Autodesk Fusion 360 part; units mm, degrees
(part 4 of 7)
  spline S257 degree 3 poles (0.768, 12.1665) (0.7347, 12.1331) (0.6728, 12.1046) (0.6299, 12.1046) knots 0 0 0 0 1 1 1 1
  spline S258 degree 3 poles (0.6299, 12.1046) (0.5918, 12.1046) (0.4775, 12.0331) (0.3775, 11.9474) knots 0 0 0 0 1 1 1 1
  spline S259 degree 3 poles (0.3775, 11.9474) (0.2727, 11.8617) (0.1298, 11.7569) (0.0584, 11.7188) knots 0 0 0 0 1 1 1 1
  spline S260 degree 3 poles (0.0584, 11.7188) (-0.0131, 11.6855) (-0.175, 11.5807) (-0.294, 11.4997) knots 0 0 0 0 1 1 1 1
  spline S261 degree 3 poles (-0.294, 11.4997) (-0.5417, 11.3235) (-0.637, 11.3045) (-0.6131, 11.4283) knots 0 0 0 0 1 1 1 1
  spline S262 degree 3 poles (-0.6131, 11.4283) (-0.5989, 11.514) (-0.5179, 11.5664) (0.4584, 12.176) knots 0 0 0 0 1 1 1 1
  spline S263 degree 3 poles (-2.9087, 11.6283) (-3.0564, 11.6283) (-3.0992, 11.6474) (-3.0992, 11.714) knots 0 0 0 0 1 1 1 1
  spline S264 degree 3 poles (-3.0992, 11.714) (-3.0992, 11.7855) (-3.0325, 11.795) (-2.5372, 11.8093) knots 0 0 0 0 1 1 1 1
  spline S265 degree 3 poles (-2.5372, 11.8093) (-2.2324, 11.8141) (-1.9324, 11.8093) (-1.8705, 11.795) knots 0 0 0 0 1 1 1 1
  spline S266 degree 3 poles (-1.8705, 11.795) (-1.68, 11.7474) (-1.7514, 11.6378) (-1.9895, 11.6045) knots 0 0 0 0 1 1 1 1
  spline S267 degree 3 poles (-1.9895, 11.6045) (-2.2229, 11.5712) (-2.4801, 11.4045) (-2.4801, 11.2806) knots 0 0 0 0 1 1 1 1
  spline S268 degree 3 poles (-2.4801, 11.2806) (-2.4801, 11.2473) (-2.4991, 11.1997) (-2.5229, 11.1759) knots 0 0 0 0 1 1 1 1
  spline S269 degree 3 poles (-2.5229, 11.1759) (-2.5468, 11.1473) (-2.7182, 10.7949) (-2.8992, 10.39) knots 0 0 0 0 1 1 1 1
  spline S270 degree 3 poles (-2.8992, 10.39) (-3.2373, 9.6423) (-3.8279, 8.4659) (-3.9184, 8.3516) knots 0 0 0 0 1 1 1 1
  spline S271 degree 3 poles (-3.9184, 8.3516) (-3.9946, 8.2659) (-4.0279, 8.3135) (-4.2137, 8.7803) knots 0 0 0 0 1 1 1 1
  spline S272 degree 3 poles (-4.2137, 8.7803) (-4.3042, 9.0089) (-4.4423, 9.3137) (-4.5185, 9.4661) knots 0 0 0 0 1 1 1 1
  line L24 (-4.5185, 9.4661) -> (-4.6566, 9.7376)
  line L25 (-4.6566, 9.7376) -> (-4.7947, 9.4089)
  spline S273 degree 3 poles (-4.7947, 9.4089) (-4.8709, 9.228) (-4.9471, 9.0755) (-4.9662, 9.066) knots 0 0 0 0 1 1 1 1
  spline S274 degree 3 poles (-4.9662, 9.066) (-4.99, 9.0565) (-5.0043, 9.0232) (-5.0043, 8.9898) knots 0 0 0 0 1 1 1 1
  spline S275 degree 3 poles (-5.0043, 8.9898) (-5.0043, 8.8946) (-5.2091, 8.4183) (-5.2662, 8.3802) knots 0 0 0 0 1 1 1 1
  spline S276 degree 3 poles (-5.2662, 8.3802) (-5.3424, 8.3278) (-5.4091, 8.4326) (-5.552, 8.8184) knots 0 0 0 0 1 1 1 1
  spline S277 degree 3 poles (-5.552, 8.8184) (-5.7091, 9.2375) (-6.0187, 9.9804) (-6.2616, 10.4996) knots 0 0 0 0 1 1 1 1
  spline S278 degree 3 poles (-6.2616, 10.4996) (-6.3569, 10.6996) (-6.4331, 10.8806) (-6.4331, 10.8949) knots 0 0 0 0 1 1 1 1
  spline S279 degree 3 poles (-6.4331, 10.8949) (-6.4331, 10.9758) (-6.695, 11.5188) (-6.7617, 11.5712) knots 0 0 0 0 1 1 1 1
  spline S280 degree 3 poles (-6.7617, 11.5712) (-6.7998, 11.5997) (-6.895, 11.6283) (-6.9712, 11.6283) knots 0 0 0 0 1 1 1 1
  spline S281 degree 3 poles (-6.9712, 11.6283) (-7.057, 11.6283) (-7.0998, 11.6474) (-7.0903, 11.6902) knots 0 0 0 0 1 1 1 1
  spline S282 degree 3 poles (-7.0903, 11.6902) (-7.076, 11.7283) (-6.9093, 11.7521) (-6.5331, 11.7617) knots 0 0 0 0 1 1 1 1
  spline S283 degree 3 poles (-6.5331, 11.7617) (-6.0425, 11.7712) (-5.9997, 11.7664) (-6.0139, 11.6902) knots 0 0 0 0 1 1 1 1
  spline S284 degree 3 poles (-6.0139, 11.6902) (-6.0235, 11.6378) (-6.0854, 11.595) (-6.1711, 11.5807) knots 0 0 0 0 1 1 1 1
  spline S285 degree 3 poles (-6.1711, 11.5807) (-6.2473, 11.5664) (-6.3045, 11.5426) (-6.2997, 11.5235) knots 0 0 0 0 1 1 1 1
  spline S286 degree 3 poles (-6.2997, 11.5235) (-6.2521, 11.3711) (-6.214, 11.2806) (-6.0901, 11.0092) knots 0 0 0 0 1 1 1 1
  spline S287 degree 3 poles (-6.0901, 11.0092) (-6.0092, 10.8377) (-5.8806, 10.552) (-5.8044, 10.3662) knots 0 0 0 0 1 1 1 1
  spline S288 degree 3 poles (-5.8044, 10.3662) (-5.7282, 10.1852) (-5.6377, 9.99) (-5.6044, 9.9376) knots 0 0 0 0 1 1 1 1
  spline S289 degree 3 poles (-5.6044, 9.9376) (-5.571, 9.8852) (-5.5043, 9.7376) (-5.4615, 9.6042) knots 0 0 0 0 1 1 1 1
  spline S290 degree 3 poles (-5.4615, 9.6042) (-5.4186, 9.4756) (-5.3519, 9.3137) (-5.3186, 9.2518) knots 0 0 0 0 1 1 1 1
  line L26 (-5.3186, 9.2518) -> (-5.2519, 9.1327)
  line L27 (-5.2519, 9.1327) -> (-5.1614, 9.3232)
  spline S291 degree 3 poles (-5.1614, 9.3232) (-5.109, 9.4232) (-5.0281, 9.609) (-4.9852, 9.728) knots 0 0 0 0 1 1 1 1
  spline S292 degree 3 poles (-4.9852, 9.728) (-4.9043, 9.9423) (-4.9043, 9.9566) (-5.0043, 10.2043) knots 0 0 0 0 1 1 1 1
  spline S293 degree 3 poles (-5.0043, 10.2043) (-5.1948, 10.6663) (-5.2519, 10.7901) (-5.3615, 11.0092) knots 0 0 0 0 1 1 1 1
  spline S294 degree 3 poles (-5.3615, 11.0092) (-5.4186, 11.1282) (-5.4853, 11.2902) (-5.4996, 11.3759) knots 0 0 0 0 1 1 1 1
  spline S295 degree 3 poles (-5.4996, 11.3759) (-5.5377, 11.5426) (-5.5996, 11.6093) (-5.7377, 11.6331) knots 0 0 0 0 1 1 1 1
  spline S296 degree 3 poles (-5.7377, 11.6331) (-5.7901, 11.6426) (-5.8377, 11.6807) (-5.852, 11.714) knots 0 0 0 0 1 1 1 1
  spline S297 degree 3 poles (-5.852, 11.714) (-5.8663, 11.7569) (-5.7425, 11.7712) (-5.3377, 11.7712) knots 0 0 0 0 1 1 1 1
  spline S298 degree 3 poles (-5.3377, 11.7712) (-4.8566, 11.7712) (-4.809, 11.7617) (-4.8233, 11.6902) knots 0 0 0 0 1 1 1 1
  spline S299 degree 3 poles (-4.8233, 11.6902) (-4.8328, 11.6378) (-4.8947, 11.595) (-4.9805, 11.5807) knots 0 0 0 0 1 1 1 1
  spline S300 degree 3 poles (-4.9805, 11.5807) (-5.0567, 11.5664) (-5.1281, 11.5235) (-5.1376, 11.4807) knots 0 0 0 0 1 1 1 1
  spline S301 degree 3 poles (-5.1376, 11.4807) (-5.1424, 11.4426) (-5.0757, 11.2425) (-4.9805, 11.0377) knots 0 0 0 0 1 1 1 1
  spline S302 degree 3 poles (-4.9805, 11.0377) (-4.89, 10.8377) (-4.8138, 10.6472) (-4.8138, 10.6186) knots 0 0 0 0 1 1 1 1
  spline S303 degree 3 poles (-4.8138, 10.6186) (-4.8138, 10.5281) (-4.6614, 10.2472) (-4.6233, 10.271) knots 0 0 0 0 1 1 1 1
  spline S304 degree 3 poles (-4.6233, 10.271) (-4.5566, 10.3091) (-4.3851, 10.7187) (-4.3851, 10.8282) knots 0 0 0 0 1 1 1 1
  spline S305 degree 3 poles (-4.3851, 10.8282) (-4.3899, 10.8901) (-4.428, 11.0235) (-4.4804, 11.1282) knots 0 0 0 0 1 1 1 1
  spline S306 degree 3 poles (-4.4804, 11.1282) (-4.5328, 11.233) (-4.5709, 11.3664) (-4.5756, 11.4283) knots 0 0 0 0 1 1 1 1
  spline S307 degree 3 poles (-4.5756, 11.4283) (-4.5756, 11.4854) (-4.609, 11.5473) (-4.6471, 11.5616) knots 0 0 0 0 1 1 1 1
  spline S308 degree 3 poles (-4.6471, 11.5616) (-4.6852, 11.5807) (-4.7185, 11.6331) (-4.7185, 11.6807) knots 0 0 0 0 1 1 1 1
  spline S309 degree 3 poles (-4.7185, 11.6807) (-4.7185, 11.7664) (-4.6757, 11.7712) (-4.1708, 11.7712) knots 0 0 0 0 1 1 1 1
  spline S310 degree 3 poles (-4.1708, 11.7712) (-3.6803, 11.7712) (-3.6231, 11.7617) (-3.6231, 11.6902) knots 0 0 0 0 1 1 1 1
  spline S311 degree 3 poles (-3.6231, 11.6902) (-3.6231, 11.6188) (-3.666, 11.6045) (-3.9041, 11.6045) knots 0 0 0 0 1 1 1 1
  spline S312 degree 3 poles (-3.9041, 11.6045) (-4.0613, 11.6045) (-4.2042, 11.5854) (-4.2232, 11.5664) knots 0 0 0 0 1 1 1 1
  spline S313 degree 3 poles (-4.2232, 11.5664) (-4.247, 11.5473) (-4.2327, 11.4616) (-4.1994, 11.3759) knots 0 0 0 0 1 1 1 1
  spline S314 degree 3 poles (-4.1994, 11.3759) (-4.1661, 11.2902) (-4.066, 11.033) (-3.9803, 10.7949) knots 0 0 0 0 1 1 1 1
  spline S315 degree 3 poles (-3.9803, 10.7949) (-3.8946, 10.5615) (-3.7565, 10.2186) (-3.6755, 10.0376) knots 0 0 0 0 1 1 1 1
  spline S316 degree 3 poles (-3.6755, 10.0376) (-3.5279, 9.7137) (-3.5231, 9.709) (-3.4517, 9.8138) knots 0 0 0 0 1 1 1 1
  spline S317 degree 3 poles (-3.4517, 9.8138) (-3.4088, 9.8709) (-3.2945, 10.1138) (-3.1945, 10.3567) knots 0 0 0 0 1 1 1 1
  spline S318 degree 3 poles (-3.1945, 10.3567) (-3.0945, 10.5996) (-2.9468, 10.9473) (-2.8659, 11.1282) knots 0 0 0 0 1 1 1 1
  spline S319 degree 3 poles (-2.8659, 11.1282) (-2.6658, 11.5807) (-2.6706, 11.6283) (-2.9087, 11.6283) knots 0 0 0 0 1 1 1 1
  spline S320 degree 3 poles (0.387, 11.6331) (0.2679, 11.6807) (0.2727, 11.6807) (0.5489, 11.8664) knots 0 0 0 0 1 1 1 1
  spline S321 degree 3 poles (0.5489, 11.8664) (0.7013, 11.9712) (0.8442, 12.0569) (0.868, 12.0569) knots 0 0 0 0 1 1 1 1
  spline S322 degree 3 poles (0.868, 12.0569) (0.8871, 12.0569) (0.9014, 11.6188) (0.9014, 11.0806) knots 0 0 0 0 1 1 1 1
  spline S323 degree 3 poles (0.9014, 11.0806) (0.9014, 10.5424) (0.9109, 10.1043) (0.9157, 10.1043) knots 0 0 0 0 1 1 1 1
  spline S324 degree 3 poles (0.9157, 10.1043) (0.9252, 10.1043) (1.049, 10.2186) (1.1919, 10.3567) knots 0 0 0 0 1 1 1 1
  spline S325 degree 3 poles (1.1919, 10.3567) (1.3348, 10.4948) (1.511, 10.6567) (1.5919, 10.7187) knots 0 0 0 0 1 1 1 1
  spline S326 degree 3 poles (1.5919, 10.7187) (1.7062, 10.8044) (1.7205, 10.833) (1.6634, 10.8711) knots 0 0 0 0 1 1 1 1
  spline S327 degree 3 poles (1.6634, 10.8711) (1.6253, 10.8949) (1.4967, 10.9092) (1.3776, 10.8996) knots 0 0 0 0 1 1 1 1
  spline S328 degree 3 poles (1.3776, 10.8996) (1.2157, 10.8949) (1.1633, 10.9092) (1.1633, 10.9615) knots 0 0 0 0 1 1 1 1
  spline S329 degree 3 poles (1.1633, 10.9615) (1.1633, 11.0187) (1.2633, 11.0377) (1.7015, 11.0473) knots 0 0 0 0 1 1 1 1
  spline S330 degree 3 poles (1.7015, 11.0473) (2.2349, 11.0616) (2.2397, 11.0568) (2.2254, 10.9568) knots 0 0 0 0 1 1 1 1
  spline S331 degree 3 poles (2.2254, 10.9568) (2.2158, 10.8853) (2.1349, 10.8091) (2.0063, 10.7425) knots 0 0 0 0 1 1 1 1
  spline S332 degree 3 poles (2.0063, 10.7425) (1.5919, 10.5234) (1.049, 10.009) (1.2347, 10.009) knots 0 0 0 0 1 1 1 1
  spline S333 degree 3 poles (1.2347, 10.009) (1.2633, 10.009) (1.2824, 9.9662) (1.2824, 9.9185) knots 0 0 0 0 1 1 1 1
  spline S334 degree 3 poles (1.2824, 9.9185) (1.2824, 9.8661) (1.3014, 9.8185) (1.3252, 9.809) knots 0 0 0 0 1 1 1 1
  spline S335 degree 3 poles (1.3252, 9.809) (1.3491, 9.8042) (1.4538, 9.6661) (1.5634, 9.5089) knots 0 0 0 0 1 1 1 1
  spline S336 degree 3 poles (1.5634, 9.5089) (1.8682, 9.0708) (2.0301, 8.9136) (2.1682, 8.9136) knots 0 0 0 0 1 1 1 1
  line L28 (2.1682, 8.9136) -> (2.292, 8.9136)
  line L29 (2.292, 8.9136) -> (2.1444, 9.0803)
  spline S337 degree 3 poles (2.1444, 9.0803) (2.0682, 9.1708) (1.9777, 9.3375) (1.9444, 9.447) knots 0 0 0 0 1 1 1 1
  spline S338 degree 3 poles (1.9444, 9.447) (1.8729, 9.7233) (1.9158, 10.1852) (2.0349, 10.4234) knots 0 0 0 0 1 1 1 1
  spline S339 degree 3 poles (2.0349, 10.4234) (2.1492, 10.6424) (2.6159, 11.0377) (2.8159, 11.0806) knots 0 0 0 0 1 1 1 1
  spline S340 degree 3 poles (2.8159, 11.0806) (3.1779, 11.1616) (3.6399, 10.8472) (3.8066, 10.4091) knots 0 0 0 0 1 1 1 1
  spline S341 degree 3 poles (3.8066, 10.4091) (3.8589, 10.2662) (3.9018, 10.1281) (3.9018, 10.1043) knots 0 0 0 0 1 1 1 1
  spline S342 degree 3 poles (3.9018, 10.1043) (3.9018, 10.0757) (3.5494, 10.0519) (3.0826, 10.0471) knots 0 0 0 0 1 1 1 1
  line L30 (3.0826, 10.0471) -> (2.2587, 10.0328)
  line L31 (2.2587, 10.0328) -> (2.2444, 9.8947)
  spline S343 degree 3 poles (2.2444, 9.8947) (2.2111, 9.628) (2.2825, 9.4423) (2.4826, 9.247) knots 0 0 0 0 1 1 1 1
  spline S344 degree 3 poles (2.4826, 9.247) (2.8493, 8.8993) (3.1207, 8.885) (3.5922, 9.1994) knots 0 0 0 0 1 1 1 1
  spline S345 degree 3 poles (3.5922, 9.1994) (3.9161, 9.4137) (3.9494, 9.4232) (3.9494, 9.3042) knots 0 0 0 0 1 1 1 1
  spline S346 degree 3 poles (3.9494, 9.3042) (3.9494, 9.1613) (3.6589, 8.8612) (3.4065, 8.7422) knots 0 0 0 0 1 1 1 1
  spline S347 degree 3 poles (3.4065, 8.7422) (3.1827, 8.6374) (3.1065, 8.6279) (2.3587, 8.6279) knots 0 0 0 0 1 1 1 1
  line L32 (2.3587, 8.6279) -> (1.5586, 8.6279)
  line L33 (1.5586, 8.6279) -> (1.5872, 8.7755)
  spline S348 degree 3 poles (1.5872, 8.7755) (1.611, 8.9041) (1.5777, 8.9755) (1.3252, 9.3089) knots 0 0 0 0 1 1 1 1
  spline S349 degree 3 poles (1.3252, 9.3089) (1.1633, 9.5232) (1.0252, 9.7233) (1.0109, 9.7566) knots 0 0 0 0 1 1 1 1
  spline S350 degree 3 poles (1.0109, 9.7566) (0.9442, 9.9281) (0.9014, 9.7709) (0.9014, 9.347) knots 0 0 0 0 1 1 1 1
  line L34 (0.9014, 9.347) -> (0.9014, 8.8708)
  line L35 (0.9014, 8.8708) -> (1.1062, 8.8565)
  spline S351 degree 3 poles (1.1062, 8.8565) (1.2681, 8.8469) (1.3062, 8.8231) (1.3062, 8.7469) knots 0 0 0 0 1 1 1 1
  spline S352 degree 3 poles (1.3062, 8.7469) (1.3062, 8.6517) (1.2729, 8.6517) (-0.4798, 8.6517) knots 0 0 0 0 1 1 1 1
  line L36 (-0.4798, 8.6517) -> (-2.2658, 8.6517)
  line L37 (-2.2658, 8.6517) -> (-2.2801, 8.7612)
  spline S353 degree 3 poles (-2.2801, 8.7612) (-2.2943, 8.866) (-2.2991, 8.866) (-2.4944, 8.7136) knots 0 0 0 0 1 1 1 1
  spline S354 degree 3 poles (-2.4944, 8.7136) (-2.6992, 8.5517) (-3.0611, 8.2516) (-3.5231, 7.8468) knots 0 0 0 0 1 1 1 1
  spline S355 degree 3 poles (-3.5231, 7.8468) (-3.6707, 7.7182) (-4.1851, 7.2229) (-4.6709, 6.7466) knots 0 0 0 0 1 1 1 1
  spline S356 degree 3 poles (-4.6709, 6.7466) (-5.5377, 5.8894) (-5.7663, 5.7131) (-5.7663, 5.9037) knots 0 0 0 0 1 1 1 1
  spline S357 degree 3 poles (-5.7663, 5.9037) (-5.7663, 5.956) (-5.5567, 6.1846) (-5.2519, 6.4704) knots 0 0 0 0 1 1 1 1
  spline S358 degree 3 poles (-5.2519, 6.4704) (-4.79, 6.9038) (-4.3661, 7.2753) (-2.742, 8.6993) knots 0 0 0 0 1 1 1 1
  spline S359 degree 3 poles (-2.742, 8.6993) (-2.442, 8.9612) (-2.0848, 9.3089) (-1.9467, 9.4708) knots 0 0 0 0 1 1 1 1
  spline S360 degree 3 poles (-1.9467, 9.4708) (-1.8086, 9.6328) (-1.4418, 10.0281) (-1.1323, 10.3567) knots 0 0 0 0 1 1 1 1
  spline S361 degree 3 poles (-1.1323, 10.3567) (-0.8275, 10.6805) (-0.575, 10.9711) (-0.575, 11.0044) knots 0 0 0 0 1 1 1 1
  spline S362 degree 3 poles (-0.575, 11.0044) (-0.575, 11.0377) (-0.7179, 11.0568) (-1.0132, 11.0568) knots 0 0 0 0 1 1 1 1
  spline S363 degree 3 poles (-1.0132, 11.0568) (-1.3513, 11.0568) (-1.4657, 11.0377) (-1.5371, 10.9758) knots 0 0 0 0 1 1 1 1
  spline S364 degree 3 poles (-1.5371, 10.9758) (-1.5847, 10.933) (-1.6704, 10.8758) (-1.7276, 10.8472) knots 0 0 0 0 1 1 1 1
  spline S365 degree 3 poles (-1.7276, 10.8472) (-1.7847, 10.8187) (-1.8752, 10.7044) (-1.9324, 10.5901) knots 0 0 0 0 1 1 1 1
  spline S366 degree 3 poles (-1.9324, 10.5901) (-2.0276, 10.3948) (-2.1467, 10.3186) (-2.1467, 10.4615) knots 0 0 0 0 1 1 1 1
  spline S367 degree 3 poles (-2.1467, 10.4615) (-2.1467, 10.4996) (-2.1229, 10.6329) (-2.0896, 10.7568) knots 0 0 0 0 1 1 1 1
  spline S368 degree 3 poles (-2.0896, 10.7568) (-2.061, 10.8853) (-2.0181, 11.0711) (-1.9943, 11.1711) knots 0 0 0 0 1 1 1 1
  line L38 (-1.9943, 11.1711) -> (-1.9467, 11.3568)
  line L39 (-1.9467, 11.3568) -> (-1.0465, 11.3283)
  spline S369 degree 3 poles (-1.0465, 11.3283) (-0.4988, 11.3092) (-0.1369, 11.3187) (-0.1226, 11.3473) knots 0 0 0 0 1 1 1 1
  spline S370 degree 3 poles (-0.1226, 11.3473) (-0.0893, 11.3997) (0.0012, 11.4045) (0.0822, 11.3473) knots 0 0 0 0 1 1 1 1
  spline S371 degree 3 poles (0.0822, 11.3473) (0.206, 11.2711) (0.0774, 11.0616) (-0.3464, 10.6424) knots 0 0 0 0 1 1 1 1
  spline S372 degree 3 poles (-0.3464, 10.6424) (-0.5798, 10.4138) (-1.0418, 9.9376) (-1.3704, 9.5899) knots 0 0 0 0 1 1 1 1
  line L40 (-1.3704, 9.5899) -> (-1.9705, 8.9612)
  line L41 (-1.9705, 8.9612) -> (-1.0227, 8.9708)
  line L42 (-1.0227, 8.9708) -> (-0.0797, 8.9851)
  line L43 (-0.0797, 8.9851) -> (-0.0369, 9.1756)
  spline S373 degree 3 poles (-0.0369, 9.1756) (0.0203, 9.4137) (0.025, 9.4185) (0.1155, 9.328) knots 0 0 0 0 1 1 1 1
  spline S374 degree 3 poles (0.1155, 9.328) (0.1584, 9.2851) (0.187, 9.1708) (0.187, 9.0565) knots 0 0 0 0 1 1 1 1
  spline S375 degree 3 poles (0.187, 9.0565) (0.187, 8.866) (0.1917, 8.8612) (0.3394, 8.8755) knots 0 0 0 0 1 1 1 1
  spline S376 degree 3 poles (0.3394, 8.8755) (0.4727, 8.8898) (0.4965, 8.9136) (0.5299, 9.0565) knots 0 0 0 0 1 1 1 1
  spline S377 degree 3 poles (0.5299, 9.0565) (0.5727, 9.247) (0.5775, 10.8377) (0.5346, 11.2854) knots 0 0 0 0 1 1 1 1
  spline S378 degree 3 poles (0.5346, 11.2854) (0.5108, 11.5521) (0.4965, 11.595) (0.387, 11.6331) knots 0 0 0 0 1 1 1 1
  spline S379 degree 3 poles (4.4876, 11.052) (4.6924, 11.0568) (4.7115, 11.0473) (4.7115, 10.9425) knots 0 0 0 0 1 1 1 1
  spline S380 degree 3 poles (4.7115, 10.9425) (4.7115, 10.7758) (4.7972, 10.7425) (4.9162, 10.8568) knots 0 0 0 0 1 1 1 1
  spline S381 degree 3 poles (4.9162, 10.8568) (5.183, 11.1044) (5.4973, 11.1663) (5.7878, 11.0282) knots 0 0 0 0 1 1 1 1
  spline S382 degree 3 poles (5.7878, 11.0282) (5.8783, 10.9854) (6.0164, 10.8711) (6.0926, 10.7758) knots 0 0 0 0 1 1 1 1
  line L44 (6.0926, 10.7758) -> (6.2355, 10.6043)
  line L45 (6.2355, 10.6043) -> (6.2403, 9.8423)
  spline S383 degree 3 poles (6.2403, 9.8423) (6.245, 8.9136) (6.2593, 8.8469) (6.4641, 8.8279) knots 0 0 0 0 1 1 1 1
  spline S384 degree 3 poles (6.4641, 8.8279) (6.5784, 8.8184) (6.6165, 8.7898) (6.6165, 8.7184) knots 0 0 0 0 1 1 1 1
  spline S385 degree 3 poles (6.6165, 8.7184) (6.6165, 8.6326) (6.5784, 8.6279) (6.045, 8.6279) knots 0 0 0 0 1 1 1 1
  spline S386 degree 3 poles (6.045, 8.6279) (5.7307, 8.6279) (5.4735, 8.6422) (5.4735, 8.666) knots 0 0 0 0 1 1 1 1
  spline S387 degree 3 poles (5.4735, 8.666) (5.4782, 8.7565) (5.5592, 8.8136) (5.7116, 8.8279) knots 0 0 0 0 1 1 1 1
  line L46 (5.7116, 8.8279) -> (5.8783, 8.8422)
  line L47 (5.8783, 8.8422) -> (5.8783, 9.6899)
  spline S388 degree 3 poles (5.8783, 9.6899) (5.8783, 10.4519) (5.8688, 10.5424) (5.7973, 10.5853) knots 0 0 0 0 1 1 1 1
  spline S389 degree 3 poles (5.7973, 10.5853) (5.7497, 10.6139) (5.7116, 10.6615) (5.7116, 10.6996) knots 0 0 0 0 1 1 1 1
  spline S390 degree 3 poles (5.7116, 10.6996) (5.7116, 10.7806) (5.4068, 10.8853) (5.2592, 10.8472) knots 0 0 0 0 1 1 1 1
  spline S391 degree 3 poles (5.2592, 10.8472) (5.202, 10.833) (5.0591, 10.7615) (4.9543, 10.6901) knots 0 0 0 0 1 1 1 1
  line L48 (4.9543, 10.6901) -> (4.7591, 10.5615)
  line L49 (4.7591, 10.5615) -> (4.7686, 9.7042)
  line L50 (4.7686, 9.7042) -> (4.7829, 8.8422)
  line L51 (4.7829, 8.8422) -> (4.9258, 8.8279)
  spline S392 degree 3 poles (4.9258, 8.8279) (5.0687, 8.8088) (5.1544, 8.7374) (5.1115, 8.666) knots 0 0 0 0 1 1 1 1
  spline S393 degree 3 poles (5.1115, 8.666) (5.0877, 8.6279) (3.9494, 8.6088) (3.9494, 8.6469) knots 0 0 0 0 1 1 1 1
  spline S394 degree 3 poles (3.9494, 8.6469) (3.9494, 8.7565) (4.0304, 8.8184) (4.1638, 8.8184) knots 0 0 0 0 1 1 1 1
  spline S395 degree 3 poles (4.1638, 8.8184) (4.2638, 8.8184) (4.3304, 8.8469) (4.3495, 8.8946) knots 0 0 0 0 1 1 1 1
  spline S396 degree 3 poles (4.3495, 8.8946) (4.3876, 8.9946) (4.3876, 10.4805) (4.3495, 10.671) knots 0 0 0 0 1 1 1 1
  spline S397 degree 3 poles (4.3495, 10.671) (4.3257, 10.7853) (4.2876, 10.8282) (4.178, 10.8568) knots 0 0 0 0 1 1 1 1
  spline S398 degree 3 poles (4.178, 10.8568) (3.8875, 10.9282) (4.0637, 11.0425) (4.4876, 11.052) knots 0 0 0 0 1 1 1 1
  circle A0 centre (0, 0) radius 14.0811
  spline S399 degree 3 poles (-5.2833, -10.8985) (-5.4134, -10.9708) (-5.5435, -11.0141) (-5.5724, -10.9925) knots 0 0 0 0 1 1 1 1
  spline S400 degree 3 poles (-5.5724, -10.9925) (-5.6013, -10.978) (-5.7024, -11.0069) (-5.8036, -11.0647) knots 0 0 0 0 1 1 1 1
  spline S401 degree 3 poles (-5.8036, -11.0647) (-6.0348, -11.1875) (-6.0348, -11.1875) (-5.9842, -11.0214) knots 0 0 0 0 1 1 1 1
  spline S402 degree 3 poles (-5.9842, -11.0214) (-5.9264, -10.8407) (-6.1359, -10.819) (-6.3527, -10.9852) knots 0 0 0 0 1 1 1 1
  spline S403 degree 3 poles (-6.3527, -10.9852) (-6.5333, -11.1225) (-7.0319, -11.1225) (-7.2342, -10.978) knots 0 0 0 0 1 1 1 1
  spline S404 degree 3 poles (-7.2342, -10.978) (-7.3859, -10.8769) (-7.3931, -10.819) (-7.3931, -9.8436) knots 0 0 0 0 1 1 1 1
  spline S405 degree 3 poles (-7.3931, -9.8436) (-7.3931, -9.0488) (-7.4148, -8.7815) (-7.5015, -8.6587) knots 0 0 0 0 1 1 1 1
  spline S406 degree 3 poles (-7.5015, -8.6587) (-7.5955, -8.5214) (-7.5955, -8.5069) (-7.4437, -8.4636) knots 0 0 0 0 1 1 1 1
  spline S407 degree 3 poles (-7.4437, -8.4636) (-7.227, -8.4058) (-6.7067, -8.4058) (-6.6489, -8.4708) knots 0 0 0 0 1 1 1 1
  spline S408 degree 3 poles (-6.6489, -8.4708) (-6.62, -8.4925) (-6.6851, -8.5936) (-6.7862, -8.6876) knots 0 0 0 0 1 1 1 1
  spline S409 degree 3 poles (-6.7862, -8.6876) (-6.9741, -8.861) (-6.9741, -8.8754) (-6.9452, -9.7208) knots 0 0 0 0 1 1 1 1
  spline S410 degree 3 poles (-6.9452, -9.7208) (-6.9235, -10.2844) (-6.8801, -10.6167) (-6.8223, -10.689) knots 0 0 0 0 1 1 1 1
  spline S411 degree 3 poles (-6.8223, -10.689) (-6.7212, -10.8118) (-6.4755, -10.8335) (-6.0998, -10.7612) knots 0 0 0 0 1 1 1 1
  line L52 (-6.0998, -10.7612) -> (-5.8758, -10.7179)
  line L53 (-5.8758, -10.7179) -> (-5.8758, -8.7093)
  line L54 (-5.8758, -8.7093) -> (-6.0781, -8.6225)
  line L55 (-6.0781, -8.6225) -> (-6.2732, -8.5431)
  line L56 (-6.2732, -8.5431) -> (-6.0565, -8.4853)
  spline S412 degree 3 poles (-6.0565, -8.4853) (-5.9408, -8.4491) (-5.6518, -8.4275) (-5.4206, -8.4347) knots 0 0 0 0 1 1 1 1
  line L57 (-5.4206, -8.4347) -> (-5.0016, -8.4419)
  line L58 (-5.0016, -8.4419) -> (-5.1894, -8.5936)
  spline S413 degree 3 poles (-5.1894, -8.5936) (-5.3773, -8.7454) (-5.3845, -8.7743) (-5.4206, -9.7352) knots 0 0 0 0 1 1 1 1
  line L59 (-5.4206, -9.7352) -> (-5.464, -10.7179)
  line L60 (-5.464, -10.7179) -> (-5.2544, -10.7468)
  line L61 (-5.2544, -10.7468) -> (-5.0449, -10.7685)
  line L62 (-5.0449, -10.7685) -> (-5.2833, -10.8985)
  spline S414 degree 3 poles (6.0388, -10.1399) (6.4289, -11.2742) (6.5662, -11.5271) (6.7541, -11.5271) knots 0 0 0 0 1 1 1 1
  spline S415 degree 3 poles (6.7541, -11.5271) (6.8624, -11.5271) (6.8624, -11.5416) (6.7685, -11.5994) knots 0 0 0 0 1 1 1 1
  spline S416 degree 3 poles (6.7685, -11.5994) (6.6312, -11.6861) (5.6341, -11.6933) (5.5836, -11.6066) knots 0 0 0 0 1 1 1 1
  spline S417 degree 3 poles (5.5836, -11.6066) (5.5619, -11.5705) (5.6052, -11.5271) (5.6847, -11.5055) knots 0 0 0 0 1 1 1 1
  spline S418 degree 3 poles (5.6847, -11.5055) (5.8003, -11.4766) (5.8292, -11.4043) (5.8292, -11.1948) knots 0 0 0 0 1 1 1 1
  spline S419 degree 3 poles (5.8292, -11.1948) (5.8292, -10.9347) (5.3018, -9.2439) (5.1862, -9.1211) knots 0 0 0 0 1 1 1 1
  spline S420 degree 3 poles (5.1862, -9.1211) (5.1067, -9.0416) (4.8321, -9.6341) (4.7382, -10.0893) knots 0 0 0 0 1 1 1 1
  spline S421 degree 3 poles (4.7382, -10.0893) (4.6154, -10.6673) (4.8683, -11.491) (5.1934, -11.5416) knots 0 0 0 0 1 1 1 1
  spline S422 degree 3 poles (5.1934, -11.5416) (5.3524, -11.5705) (5.3451, -11.5777) (5.1573, -11.6283) knots 0 0 0 0 1 1 1 1
  spline S423 degree 3 poles (5.1573, -11.6283) (5.0489, -11.6644) (4.6732, -11.6644) (4.3264, -11.6355) knots 0 0 0 0 1 1 1 1
  spline S424 degree 3 poles (4.3264, -11.6355) (3.8206, -11.5922) (3.7339, -11.5705) (3.8784, -11.5127) knots 0 0 0 0 1 1 1 1
  spline S425 degree 3 poles (3.8784, -11.5127) (4.2324, -11.3826) (4.3191, -11.2381) (4.2686, -10.8841) knots 0 0 0 0 1 1 1 1
  spline S426 degree 3 poles (4.2686, -10.8841) (4.218, -10.5373) (3.9362, -9.6919) (3.7556, -9.3306) knots 0 0 0 0 1 1 1 1
  line L63 (3.7556, -9.3306) -> (3.6472, -9.1283)
  line L64 (3.6472, -9.1283) -> (3.5316, -9.2945)
  spline S427 degree 3 poles (3.5316, -9.2945) (3.4738, -9.3812) (3.2498, -9.9014) (3.0475, -10.4361) knots 0 0 0 0 1 1 1 1
  spline S428 degree 3 poles (3.0475, -10.4361) (2.6356, -11.5127) (2.6356, -11.5055) (3.1559, -11.5344) knots 0 0 0 0 1 1 1 1
  spline S429 degree 3 poles (3.1559, -11.5344) (3.4015, -11.5416) (3.4015, -11.5488) (3.0836, -11.6066) knots 0 0 0 0 1 1 1 1
  spline S430 degree 3 poles (3.0836, -11.6066) (2.903, -11.6355) (2.5128, -11.6644) (2.2166, -11.6644) knots 0 0 0 0 1 1 1 1
  line L65 (2.2166, -11.6644) -> (1.6747, -11.6716)
  line L66 (1.6747, -11.6716) -> (1.9564, -11.5055)
  spline S431 degree 3 poles (1.9564, -11.5055) (2.2527, -11.332) (2.5056, -10.8913) (3.3004, -9.1283) knots 0 0 0 0 1 1 1 1
  spline S432 degree 3 poles (3.3004, -9.1283) (3.5099, -8.6587) (3.705, -8.2757) (3.7339, -8.2757) knots 0 0 0 0 1 1 1 1
  spline S433 degree 3 poles (3.7339, -8.2757) (3.7628, -8.2757) (3.9073, -8.5431) (4.0518, -8.8754) knots 0 0 0 0 1 1 1 1
  spline S434 degree 3 poles (4.0518, -8.8754) (4.5431, -9.9881) (4.5648, -10.0026) (4.7454, -9.4173) knots 0 0 0 0 1 1 1 1
  spline S435 degree 3 poles (4.7454, -9.4173) (4.9116, -8.9043) (5.1862, -8.2757) (5.2512, -8.2757) knots 0 0 0 0 1 1 1 1
  spline S436 degree 3 poles (5.2512, -8.2757) (5.3307, -8.2757) (5.6414, -9.0055) (6.0388, -10.1399) knots 0 0 0 0 1 1 1 1
  spline S437 degree 3 poles (-3.1735, -8.6587) (-2.6244, -9.085) (-2.4366, -10.0459) (-2.8267, -10.4795) knots 0 0 0 0 1 1 1 1
  spline S438 degree 3 poles (-2.8267, -10.4795) (-3.123, -10.819) (-3.3108, -10.9563) (-3.6143, -11.0647) knots 0 0 0 0 1 1 1 1
  spline S439 degree 3 poles (-3.6143, -11.0647) (-3.9539, -11.1803) (-4.055, -11.1875) (-4.3657, -11.0864) knots 0 0 0 0 1 1 1 1
  spline S440 degree 3 poles (-4.3657, -11.0864) (-4.6692, -10.9852) (-4.9365, -10.7468) (-4.9365, -10.5878) knots 0 0 0 0 1 1 1 1
  spline S441 degree 3 poles (-4.9365, -10.5878) (-4.9365, -10.3422) (-4.6764, -10.2121) (-4.055, -10.1471) knots 0 0 0 0 1 1 1 1
  spline S442 degree 3 poles (-4.055, -10.1471) (-3.0218, -10.0315) (-3.0363, -10.0387) (-3.0868, -9.7208) knots 0 0 0 0 1 1 1 1
  spline S443 degree 3 poles (-3.0868, -9.7208) (-3.1952, -9.0127) (-3.4264, -8.8176) (-4.1128, -8.8249) knots 0 0 0 0 1 1 1 1
  spline S444 degree 3 poles (-4.1128, -8.8249) (-4.4308, -8.8249) (-4.6331, -8.8754) (-4.8209, -8.9838) knots 0 0 0 0 1 1 1 1
  spline S445 degree 3 poles (-4.8209, -8.9838) (-5.1388, -9.1717) (-5.1605, -9.085) (-4.8643, -8.796) knots 0 0 0 0 1 1 1 1
  spline S446 degree 3 poles (-4.8643, -8.796) (-4.4308, -8.3624) (-3.6504, -8.2974) (-3.1735, -8.6587) knots 0 0 0 0 1 1 1 1
  spline S447 degree 3 poles (1.9131, -10.4578) (1.9564, -10.978) (1.8914, -11.0141) (0.8943, -11.043) knots 0 0 0 0 1 1 1 1
  spline S448 degree 3 poles (0.8943, -11.043) (0.4102, -11.0503) (-0.0594, -11.0719) (-0.1461, -11.0792) knots 0 0 0 0 1 1 1 1
  spline S449 degree 3 poles (-0.1461, -11.0792) (-0.2328, -11.0864) (-0.3195, -11.0647) (-0.3484, -11.0286) knots 0 0 0 0 1 1 1 1
  spline S450 degree 3 poles (-0.3484, -11.0286) (-0.3701, -10.9925) (-0.0667, -10.5589) (0.3235, -10.0676) knots 0 0 0 0 1 1 1 1
  spline S451 degree 3 poles (0.3235, -10.0676) (0.7137, -9.5763) (1.1255, -9.0561) (1.2339, -8.9116) knots 0 0 0 0 1 1 1 1
  line L67 (1.2339, -8.9116) -> (1.4362, -8.637)
  line L68 (1.4362, -8.637) -> (0.8654, -8.637)
  spline S452 degree 3 poles (0.8654, -8.637) (0.2151, -8.637) (0.0562, -8.7165) (-0.1678, -9.1283) knots 0 0 0 0 1 1 1 1
  spline S453 degree 3 poles (-0.1678, -9.1283) (-0.2906, -9.374) (-0.3051, -9.3812) (-0.3123, -9.215) knots 0 0 0 0 1 1 1 1
  spline S454 degree 3 poles (-0.3123, -9.215) (-0.3123, -9.1139) (-0.2545, -8.8971) (-0.1895, -8.7309) knots 0 0 0 0 1 1 1 1
  line L69 (-0.1895, -8.7309) -> (-0.0594, -8.4202)
  line L70 (-0.0594, -8.4202) -> (1.075, -8.4202)
  spline S455 degree 3 poles (1.075, -8.4202) (1.8914, -8.4202) (2.2166, -8.4419) (2.2166, -8.5069) knots 0 0 0 0 1 1 1 1
  spline S456 degree 3 poles (2.2166, -8.5069) (2.2166, -8.6153) (1.7469, -9.215) (1.0027, -10.0676) knots 0 0 0 0 1 1 1 1
  spline S457 degree 3 poles (1.0027, -10.0676) (0.3163, -10.8552) (0.3235, -10.8985) (1.0894, -10.8263) knots 0 0 0 0 1 1 1 1
  spline S458 degree 3 poles (1.0894, -10.8263) (1.5663, -10.7829) (1.5735, -10.7757) (1.7325, -10.4867) knots 0 0 0 0 1 1 1 1
  line L71 (1.7325, -10.4867) -> (1.8914, -10.1904)
  line L72 (1.8914, -10.1904) -> (1.9131, -10.4578)
  spline S459 degree 3 poles (-0.4279, -11.7078) (-0.1245, -11.7945) (-0.1389, -11.8378) (-0.4929, -11.9173) knots 0 0 0 0 1 1 1 1
  spline S460 degree 3 poles (-0.4929, -11.9173) (-0.7675, -11.9896) (-0.8903, -12.0907) (-0.8903, -12.2569) knots 0 0 0 0 1 1 1 1
  spline S461 degree 3 poles (-0.8903, -12.2569) (-0.8903, -12.4086) (-1.071, -12.4447) (-1.1505, -12.3075) knots 0 0 0 0 1 1 1 1
  spline S462 degree 3 poles (-1.1505, -12.3075) (-1.1794, -12.2641) (-1.1938, -11.6572) (-1.1866, -10.9708) knots 0 0 0 0 1 1 1 1
  line L73 (-1.1866, -10.9708) -> (-1.1721, -9.7136)
  line L74 (-1.1721, -9.7136) -> (-1.3455, -9.8292)
  spline S463 degree 3 poles (-1.3455, -9.8292) (-1.4395, -9.887) (-1.6707, -10.1326) (-1.8513, -10.3711) knots 0 0 0 0 1 1 1 1
  line L75 (-1.8513, -10.3711) -> (-2.1837, -10.7974)
  line L76 (-2.1837, -10.7974) -> (-1.9236, -10.819)
  spline S464 degree 3 poles (-1.9236, -10.819) (-1.7791, -10.8335) (-1.649, -10.8841) (-1.6273, -10.9347) knots 0 0 0 0 1 1 1 1
  spline S465 degree 3 poles (-1.6273, -10.9347) (-1.6056, -10.9997) (-1.7502, -11.0214) (-2.1837, -11.0214) knots 0 0 0 0 1 1 1 1
  spline S466 degree 3 poles (-2.1837, -11.0214) (-2.5088, -11.0214) (-2.7689, -10.9925) (-2.7689, -10.9563) knots 0 0 0 0 1 1 1 1
  spline S467 degree 3 poles (-2.7689, -10.9563) (-2.7689, -10.9202) (-2.5883, -10.7323) (-2.3715, -10.5517) knots 0 0 0 0 1 1 1 1
  spline S468 degree 3 poles (-2.3715, -10.5517) (-2.1548, -10.3639) (-1.9958, -10.1832) (-2.0175, -10.1471) knots 0 0 0 0 1 1 1 1
  spline S469 degree 3 poles (-2.0175, -10.1471) (-2.0392, -10.111) (-2.0175, -10.0893) (-1.9669, -10.0965) knots 0 0 0 0 1 1 1 1
  spline S470 degree 3 poles (-1.9669, -10.0965) (-1.9163, -10.111) (-1.8296, -10.0315) (-1.7646, -9.9231) knots 0 0 0 0 1 1 1 1
  spline S471 degree 3 poles (-1.7646, -9.9231) (-1.649, -9.728) (-1.649, -9.7208) (-2.1186, -9.2439) knots 0 0 0 0 1 1 1 1
  spline S472 degree 3 poles (-2.1186, -9.2439) (-2.3788, -8.9838) (-2.7183, -8.702) (-2.8773, -8.6153) knots 0 0 0 0 1 1 1 1
  line L77 (-2.8773, -8.6153) -> (-3.1663, -8.4564)
  line L78 (-3.1663, -8.4564) -> (-2.5955, -8.4347)
  spline S473 degree 3 poles (-2.5955, -8.4347) (-1.9814, -8.413) (-1.9091, -8.4347) (-2.0392, -8.5936) knots 0 0 0 0 1 1 1 1
  spline S474 degree 3 poles (-2.0392, -8.5936) (-2.1042, -8.6731) (-2.0319, -8.7743) (-1.6707, -9.1283) knots 0 0 0 0 1 1 1 1
  line L79 (-1.6707, -9.1283) -> (-1.2155, -9.5691)
  line L80 (-1.2155, -9.5691) -> (-1.1721, -9.3306)
  spline S475 degree 3 poles (-1.1721, -9.3306) (-1.0999, -8.8899) (-1.1721, -8.5936) (-1.3817, -8.5142) knots 0 0 0 0 1 1 1 1
  spline S476 degree 3 poles (-1.3817, -8.5142) (-1.5478, -8.4491) (-1.4756, -8.4347) (-0.9843, -8.4275) knots 0 0 0 0 1 1 1 1
  spline S477 degree 3 poles (-0.9843, -8.4275) (-0.399, -8.4202) (-0.1967, -8.4997) (-0.5652, -8.5936) knots 0 0 0 0 1 1 1 1
  line L81 (-0.5652, -8.5936) -> (-0.7458, -8.637)
  line L82 (-0.7458, -8.637) -> (-0.7314, -10.1326)
  line L83 (-0.7314, -10.1326) -> (-0.7097, -11.6283)
  line L84 (-0.7097, -11.6283) -> (-0.4279, -11.7078)
  spline S478 degree 3 poles (3.2862, -4.7869) (3.2932, -4.78) (3.4519, -4.7635) (3.5898, -4.7557) knots 0 0 0 0 1 1 1 1
  spline S479 degree 3 poles (3.5898, -4.7557) (3.6592, -4.7523) (3.739, -4.7427) (3.7676, -4.7358) knots 0 0 0 0 1 1 1 1
  spline S480 degree 3 poles (3.7676, -4.7358) (3.7963, -4.728) (3.8466, -4.7184) (3.8804, -4.7132) knots 0 0 0 0 1 1 1 1
  spline S481 degree 3 poles (3.8804, -4.7132) (4.027, -4.6915) (4.2742, -4.6213) (4.3028, -4.5926) knots 0 0 0 0 1 1 1 1
  spline S482 degree 3 poles (4.3028, -4.5926) (4.3185, -4.577) (4.3211, -4.0783) (4.3054, -3.9707) knots 0 0 0 0 1 1 1 1
  spline S483 degree 3 poles (4.3054, -3.9707) (4.2872, -3.8406) (4.2577, -3.661) (4.2534, -3.6532) knots 0 0 0 0 1 1 1 1
  spline S484 degree 3 poles (4.2534, -3.6532) (4.2508, -3.6498) (4.243, -3.6142) (4.2361, -3.5743) knots 0 0 0 0 1 1 1 1
  spline S485 degree 3 poles (4.2361, -3.5743) (4.2152, -3.4633) (4.1658, -3.3045) (4.1276, -3.2299) knots 0 0 0 0 1 1 1 1
  spline S486 degree 3 poles (4.1276, -3.2299) (4.1181, -3.2108) (4.099, -3.1675) (4.0851, -3.1319) knots 0 0 0 0 1 1 1 1
  spline S487 degree 3 poles (4.0851, -3.1319) (4.0461, -3.0339) (3.9576, -2.8535) (3.8952, -2.7442) knots 0 0 0 0 1 1 1 1
  spline S488 degree 3 poles (3.8952, -2.7442) (3.8284, -2.6279) (3.8232, -2.5976) (3.844, -2.4727) knots 0 0 0 0 1 1 1 1
  spline S489 degree 3 poles (3.844, -2.4727) (3.8665, -2.3426) (3.8752, -2.2723) (3.89, -2.0884) knots 0 0 0 0 1 1 1 1
  spline S490 degree 3 poles (3.89, -2.0884) (3.9004, -1.9652) (3.9082, -1.908) (3.9186, -1.8906) knots 0 0 0 0 1 1 1 1
  spline S491 degree 3 poles (3.9186, -1.8906) (3.9325, -1.8655) (4.0365, -1.7831) (4.0756, -1.7666) knots 0 0 0 0 1 1 1 1
  spline S492 degree 3 poles (4.0756, -1.7666) (4.0947, -1.7579) (4.1484, -1.7189) (4.1901, -1.6807) knots 0 0 0 0 1 1 1 1
  spline S493 degree 3 poles (4.1901, -1.6807) (4.1988, -1.6738) (4.2109, -1.6677) (4.217, -1.6677) knots 0 0 0 0 1 1 1 1
  spline S494 degree 3 poles (4.217, -1.6677) (4.2239, -1.6677) (4.2361, -1.6599) (4.2447, -1.6504) knots 0 0 0 0 1 1 1 1
  spline S495 degree 3 poles (4.2447, -1.6504) (4.2534, -1.6408) (4.2638, -1.633) (4.2681, -1.633) knots 0 0 0 0 1 1 1 1
  spline S496 degree 3 poles (4.2681, -1.633) (4.276, -1.633) (4.4225, -1.5367) (4.4659, -1.5038) knots 0 0 0 0 1 1 1 1
  spline S497 degree 3 poles (4.4659, -1.5038) (4.5431, -1.4448) (4.6385, -1.378) (4.6672, -1.3632) knots 0 0 0 0 1 1 1 1
  spline S498 degree 3 poles (4.6672, -1.3632) (4.6854, -1.3537) (4.7496, -1.3103) (4.8112, -1.2661) knots 0 0 0 0 1 1 1 1
  spline S499 degree 3 poles (4.8112, -1.2661) (4.9066, -1.1976) (4.9656, -1.1568) (5.0644, -1.0926) knots 0 0 0 0 1 1 1 1
  spline S500 degree 3 poles (5.0644, -1.0926) (5.0766, -1.0848) (5.1052, -1.0648) (5.1295, -1.0475) knots 0 0 0 0 1 1 1 1
  spline S501 degree 3 poles (5.1295, -1.0475) (5.1529, -1.0301) (5.192, -1.0033) (5.2162, -0.9868) knots 0 0 0 0 1 1 1 1
  spline S502 degree 3 poles (5.2162, -0.9868) (5.3897, -0.8688) (5.545, -0.7508) (5.6231, -0.678) knots 0 0 0 0 1 1 1 1
  spline S503 degree 3 poles (5.6231, -0.678) (5.6786, -0.6259) (5.6734, -0.6173) (5.5528, -0.5557) knots 0 0 0 0 1 1 1 1
  spline S504 degree 3 poles (5.5528, -0.5557) (5.4522, -0.5045) (5.4027, -0.4776) (5.3203, -0.429) knots 0 0 0 0 1 1 1 1
  spline S505 degree 3 poles (5.3203, -0.429) (5.2917, -0.4125) (5.2431, -0.3857) (5.2119, -0.3683) knots 0 0 0 0 1 1 1 1
  spline S506 degree 3 poles (5.2119, -0.3683) (5.0974, -0.3067) (4.9577, -0.2252) (4.8788, -0.1731) knots 0 0 0 0 1 1 1 1
  spline S507 degree 3 poles (4.8788, -0.1731) (4.8337, -0.1436) (4.7747, -0.1055) (4.747, -0.089) knots 0 0 0 0 1 1 1 1
  spline S508 degree 3 poles (4.747, -0.089) (4.7192, -0.0725) (4.6732, -0.0378) (4.6437, -0.0135) knots 0 0 0 0 1 1 1 1
  spline S509 degree 3 poles (4.6437, -0.0135) (4.6151, 0.0116) (4.5882, 0.0324) (4.583, 0.0324) knots 0 0 0 0 1 1 1 1
  spline S510 degree 3 poles (4.583, 0.0324) (4.557, 0.0324) (4.1623, 0.4297) (4.1623, 0.4557) knots 0 0 0 0 1 1 1 1
  spline S511 degree 3 poles (4.1623, 0.4557) (4.1623, 0.4644) (4.1571, 0.4766) (4.151, 0.4818) knots 0 0 0 0 1 1 1 1
  spline S512 degree 3 poles (4.151, 0.4818) (4.1432, 0.4904) (4.1398, 0.6119) (4.1354, 1.0022) knots 0 0 0 0 1 1 1 1
  spline S513 degree 3 poles (4.1354, 1.0022) (4.1328, 1.2824) (4.1259, 1.6363) (4.1207, 1.7881) knots 0 0 0 0 1 1 1 1
  spline S514 degree 3 poles (4.1207, 1.7881) (4.1094, 2.1108) (4.1094, 2.1099) (4.0452, 2.0631) knots 0 0 0 0 1 1 1 1
  spline S515 degree 3 poles (4.0452, 2.0631) (4.0235, 2.0475) (3.9958, 2.0345) (3.9828, 2.0336) knots 0 0 0 0 1 1 1 1
  spline S516 degree 3 poles (3.9828, 2.0336) (3.9585, 2.0318) (3.9585, 2.0327) (3.9593, 2.0796) knots 0 0 0 0 1 1 1 1
  spline S517 degree 3 poles (3.9593, 2.0796) (3.9602, 2.1307) (3.9567, 2.1221) (4.0973, 2.4005) knots 0 0 0 0 1 1 1 1
  spline S518 degree 3 poles (4.0973, 2.4005) (4.1346, 2.4742) (4.1779, 2.5653) (4.1935, 2.6017) knots 0 0 0 0 1 1 1 1
  spline S519 degree 3 poles (4.1935, 2.6017) (4.2092, 2.639) (4.243, 2.7006) (4.2673, 2.7397) knots 0 0 0 0 1 1 1 1
  spline S520 degree 3 poles (4.2673, 2.7397) (4.3028, 2.7952) (4.3107, 2.8134) (4.3037, 2.8247) knots 0 0 0 0 1 1 1 1
  spline S521 degree 3 poles (4.3037, 2.8247) (4.2959, 2.8368) (4.2655, 2.8386) (4.0218, 2.8368) knots 0 0 0 0 1 1 1 1
  spline S522 degree 3 poles (4.0218, 2.8368) (3.7902, 2.8359) (3.7442, 2.8333) (3.7217, 2.8221) knots 0 0 0 0 1 1 1 1
  spline S523 degree 3 poles (3.7217, 2.8221) (3.7069, 2.8143) (3.6878, 2.8082) (3.6792, 2.8082) knots 0 0 0 0 1 1 1 1
  spline S524 degree 3 poles (3.6792, 2.8082) (3.6592, 2.8082) (3.5603, 2.7778) (3.4814, 2.7475) knots 0 0 0 0 1 1 1 1
  spline S525 degree 3 poles (3.4814, 2.7475) (3.412, 2.7206) (3.3487, 2.6798) (3.2064, 2.5723) knots 0 0 0 0 1 1 1 1
  spline S526 degree 3 poles (3.2064, 2.5723) (3.1518, 2.5306) (3.0963, 2.4925) (3.0841, 2.4881) knots 0 0 0 0 1 1 1 1
  spline S527 degree 3 poles (3.0841, 2.4881) (3.0598, 2.4786) (3.0486, 2.4898) (3.026, 2.548) knots 0 0 0 0 1 1 1 1
  spline S528 degree 3 poles (3.026, 2.548) (3.0061, 2.6) (2.9497, 2.692) (2.8976, 2.7579) knots 0 0 0 0 1 1 1 1
  spline S529 degree 3 poles (2.8976, 2.7579) (2.8699, 2.7926) (2.8386, 2.8368) (2.8274, 2.8559) knots 0 0 0 0 1 1 1 1
  spline S530 degree 3 poles (2.8274, 2.8559) (2.8005, 2.9019) (2.6964, 3.0077) (2.679, 3.0077) knots 0 0 0 0 1 1 1 1
  spline S531 degree 3 poles (2.679, 3.0077) (2.6712, 3.0077) (2.6409, 3.0285) (2.6122, 3.0537) knots 0 0 0 0 1 1 1 1
  spline S532 degree 3 poles (2.6122, 3.0537) (2.5827, 3.078) (2.5307, 3.1118) (2.496, 3.1283) knots 0 0 0 0 1 1 1 1
  spline S533 degree 3 poles (2.496, 3.1283) (2.4604, 3.1439) (2.4257, 3.1604) (2.4188, 3.1647) knots 0 0 0 0 1 1 1 1
  spline S534 degree 3 poles (2.4188, 3.1647) (2.4119, 3.169) (2.3919, 3.1794) (2.3754, 3.1881) knots 0 0 0 0 1 1 1 1
  spline S535 degree 3 poles (2.3754, 3.1881) (2.359, 3.1977) (2.3173, 3.2202) (2.2844, 3.2393) knots 0 0 0 0 1 1 1 1
  spline S536 degree 3 poles (2.2844, 3.2393) (2.2505, 3.2584) (2.208, 3.2827) (2.1889, 3.2931) knots 0 0 0 0 1 1 1 1
  spline S537 degree 3 poles (2.1889, 3.2931) (2.1699, 3.3044) (2.1464, 3.32) (2.1369, 3.3278) knots 0 0 0 0 1 1 1 1
  spline S538 degree 3 poles (2.1369, 3.3278) (2.1274, 3.3365) (2.0736, 3.3659) (2.0172, 3.3937) knots 0 0 0 0 1 1 1 1
  spline S539 degree 3 poles (2.0172, 3.3937) (1.9608, 3.4215) (1.9096, 3.4518) (1.9027, 3.4622) knots 0 0 0 0 1 1 1 1
  spline S540 degree 3 poles (1.9027, 3.4622) (1.8958, 3.4718) (1.8897, 3.4935) (1.8897, 3.5091) knots 0 0 0 0 1 1 1 1
  line L85 (1.8897, 3.5091) -> (1.8897, 3.5386)
  line L86 (1.8897, 3.5386) -> (1.9565, 3.5334)
  spline S541 degree 3 poles (1.9565, 3.5334) (1.9938, 3.5308) (2.0536, 3.5273) (2.0892, 3.5255) knots 0 0 0 0 1 1 1 1
  spline S542 degree 3 poles (2.0892, 3.5255) (2.1673, 3.5212) (2.3728, 3.4961) (2.3832, 3.49) knots 0 0 0 0 1 1 1 1
  spline S543 degree 3 poles (2.3832, 3.49) (2.3867, 3.4874) (2.4231, 3.4787) (2.463, 3.4718) knots 0 0 0 0 1 1 1 1
  spline S544 degree 3 poles (2.463, 3.4718) (2.5029, 3.464) (2.5619, 3.4518) (2.594, 3.4449) knots 0 0 0 0 1 1 1 1
  spline S545 degree 3 poles (2.594, 3.4449) (2.6261, 3.4379) (2.6903, 3.4327) (2.7371, 3.4327) knots 0 0 0 0 1 1 1 1
  line L87 (2.7371, 3.4327) -> (2.8222, 3.4327)
  line L88 (2.8222, 3.4327) -> (2.9271, 3.5386)
  spline S546 degree 3 poles (2.9271, 3.5386) (2.9844, 3.5975) (3.0859, 3.6982) (3.1518, 3.7624) knots 0 0 0 0 1 1 1 1
  spline S547 degree 3 poles (3.1518, 3.7624) (3.314, 3.9211) (3.3383, 3.9523) (3.3383, 4.0044) knots 0 0 0 0 1 1 1 1
  spline S548 degree 3 poles (3.3383, 4.0044) (3.3383, 4.0642) (3.3131, 4.0972) (3.1145, 4.301) knots 0 0 0 0 1 1 1 1
  spline S549 degree 3 poles (3.1145, 4.301) (2.993, 4.4251) (2.915, 4.4971) (2.8586, 4.537) knots 0 0 0 0 1 1 1 1
  spline S550 degree 3 poles (2.8586, 4.537) (2.8144, 4.5691) (2.7727, 4.6046) (2.7658, 4.6168) knots 0 0 0 0 1 1 1 1
  spline S551 degree 3 poles (2.7658, 4.6168) (2.7554, 4.6358) (2.7562, 4.6402) (2.771, 4.6567) knots 0 0 0 0 1 1 1 1
  spline S552 degree 3 poles (2.771, 4.6567) (2.7953, 4.6836) (2.9315, 4.7824) (3.0026, 4.8249) knots 0 0 0 0 1 1 1 1
  spline S553 degree 3 poles (3.0026, 4.8249) (3.1379, 4.9047) (3.3079, 5.0279) (3.438, 5.1398) knots 0 0 0 0 1 1 1 1
  spline S554 degree 3 poles (3.438, 5.1398) (3.4901, 5.1849) (3.5465, 5.2335) (3.5621, 5.2465) knots 0 0 0 0 1 1 1 1
  spline S555 degree 3 poles (3.5621, 5.2465) (3.5785, 5.2604) (3.5968, 5.2717) (3.6028, 5.2717) knots 0 0 0 0 1 1 1 1
  spline S556 degree 3 poles (3.6028, 5.2717) (3.6089, 5.2717) (3.6158, 5.2769) (3.6184, 5.2829) knots 0 0 0 0 1 1 1 1
  spline S557 degree 3 poles (3.6184, 5.2829) (3.6211, 5.2899) (3.6436, 5.3055) (3.6688, 5.3194) knots 0 0 0 0 1 1 1 1
  spline S558 degree 3 poles (3.6688, 5.3194) (3.7303, 5.3515) (3.9177, 5.4634) (3.9724, 5.5015) knots 0 0 0 0 1 1 1 1
  spline S559 degree 3 poles (3.9724, 5.5015) (3.9966, 5.518) (4.0357, 5.5388) (4.0582, 5.5466) knots 0 0 0 0 1 1 1 1
  spline S560 degree 3 poles (4.0582, 5.5466) (4.0817, 5.5544) (4.1129, 5.5718) (4.1285, 5.5848) knots 0 0 0 0 1 1 1 1
  line L89 (4.1285, 5.5848) -> (4.1563, 5.6074)
  line L90 (4.1563, 5.6074) -> (4.1207, 5.6455)
  spline S561 degree 3 poles (4.1207, 5.6455) (4.099, 5.6698) (4.0556, 5.7002) (4.0045, 5.7262) knots 0 0 0 0 1 1 1 1
  spline S562 degree 3 poles (4.0045, 5.7262) (3.9567, 5.7514) (3.8761, 5.806) (3.8067, 5.8615) knots 0 0 0 0 1 1 1 1
  spline S563 degree 3 poles (3.8067, 5.8615) (3.7425, 5.9127) (3.6523, 5.9804) (3.6072, 6.0107) knots 0 0 0 0 1 1 1 1
  spline S564 degree 3 poles (3.6072, 6.0107) (3.5621, 6.0419) (3.4944, 6.0879) (3.4571, 6.1139) knots 0 0 0 0 1 1 1 1
  spline S565 degree 3 poles (3.4571, 6.1139) (3.4207, 6.14) (3.3834, 6.1642) (3.3747, 6.1694) knots 0 0 0 0 1 1 1 1
  spline S566 degree 3 poles (3.3747, 6.1694) (3.3669, 6.1738) (3.327, 6.1981) (3.2862, 6.2224) knots 0 0 0 0 1 1 1 1
  spline S567 degree 3 poles (3.2862, 6.2224) (3.2038, 6.2718) (3.0451, 6.3473) (3.0234, 6.3473) knots 0 0 0 0 1 1 1 1
  spline S568 degree 3 poles (3.0234, 6.3473) (3.0165, 6.3473) (3.0078, 6.3507) (3.0043, 6.3551) knots 0 0 0 0 1 1 1 1
  spline S569 degree 3 poles (3.0043, 6.3551) (2.9991, 6.3646) (2.8751, 6.4028) (2.8265, 6.4115) knots 0 0 0 0 1 1 1 1
  spline S570 degree 3 poles (2.8265, 6.4115) (2.81, 6.4141) (2.7025, 6.4201) (2.588, 6.4253) knots 0 0 0 0 1 1 1 1
  spline S571 degree 3 poles (2.588, 6.4253) (2.3217, 6.4366) (2.3321, 6.4349) (2.3321, 6.48) knots 0 0 0 0 1 1 1 1
  spline S572 degree 3 poles (2.3321, 6.48) (2.3321, 6.4999) (2.3399, 6.532) (2.3485, 6.5511) knots 0 0 0 0 1 1 1 1
  spline S573 degree 3 poles (2.3485, 6.5511) (2.3581, 6.5702) (2.3737, 6.6075) (2.3824, 6.6335) knots 0 0 0 0 1 1 1 1
  spline S574 degree 3 poles (2.3824, 6.6335) (2.4049, 6.6977) (2.4171, 6.7307) (2.4422, 6.8027) knots 0 0 0 0 1 1 1 1
  spline S575 degree 3 poles (2.4422, 6.8027) (2.4604, 6.8538) (2.4639, 6.8799) (2.4648, 6.9675) knots 0 0 0 0 1 1 1 1
  spline S576 degree 3 poles (2.4648, 6.9675) (2.4648, 7.0455) (2.4613, 7.0811) (2.4509, 7.1097) knots 0 0 0 0 1 1 1 1
  spline S577 degree 3 poles (2.4509, 7.1097) (2.4431, 7.1306) (2.4362, 7.1583) (2.4362, 7.1713) knots 0 0 0 0 1 1 1 1
  spline S578 degree 3 poles (2.4362, 7.1713) (2.4362, 7.1852) (2.4197, 7.2277) (2.3997, 7.2667) knots 0 0 0 0 1 1 1 1
  spline S579 degree 3 poles (2.3997, 7.2667) (2.3312, 7.4012) (2.228, 7.4784) (2.0267, 7.5443) knots 0 0 0 0 1 1 1 1
  spline S580 degree 3 poles (2.0267, 7.5443) (1.9244, 7.5781) (1.8402, 7.5964) (1.7821, 7.5964) knots 0 0 0 0 1 1 1 1
  spline S581 degree 3 poles (1.7821, 7.5964) (1.691, 7.5964) (1.5444, 7.5452) (1.4681, 7.4871) knots 0 0 0 0 1 1 1 1
  spline S582 degree 3 poles (1.4681, 7.4871) (1.4473, 7.4706) (1.4265, 7.4576) (1.4213, 7.4576) knots 0 0 0 0 1 1 1 1
  spline S583 degree 3 poles (1.4213, 7.4576) (1.4169, 7.4576) (1.39, 7.4272) (1.3614, 7.3908) knots 0 0 0 0 1 1 1 1
  spline S584 degree 3 poles (1.3614, 7.3908) (1.3319, 7.3535) (1.2929, 7.3032) (1.2738, 7.2797) knots 0 0 0 0 1 1 1 1
  spline S585 degree 3 poles (1.2738, 7.2797) (1.214, 7.2051) (1.1402, 7.0429) (1.1133, 6.9241) knots 0 0 0 0 1 1 1 1
  spline S586 degree 3 poles (1.1133, 6.9241) (1.0856, 6.8027) (1.0821, 6.794) (1.0483, 6.7766) knots 0 0 0 0 1 1 1 1
  spline S587 degree 3 poles (1.0483, 6.7766) (1.004, 6.7541) (0.9745, 6.7593) (0.9338, 6.8009) knots 0 0 0 0 1 1 1 1
  spline S588 degree 3 poles (0.9338, 6.8009) (0.8869, 6.8478) (0.8193, 6.9024) (0.8089, 6.9024) knots 0 0 0 0 1 1 1 1
  spline S589 degree 3 poles (0.8089, 6.9024) (0.8037, 6.9024) (0.7855, 6.9102) (0.7664, 6.9198) knots 0 0 0 0 1 1 1 1
  spline S590 degree 3 poles (0.7664, 6.9198) (0.7473, 6.9293) (0.7265, 6.9371) (0.7187, 6.9371) knots 0 0 0 0 1 1 1 1
  spline S591 degree 3 poles (0.7187, 6.9371) (0.7109, 6.9371) (0.7013, 6.9406) (0.6961, 6.9449) knots 0 0 0 0 1 1 1 1
  spline S592 degree 3 poles (0.6961, 6.9449) (0.6918, 6.9493) (0.6571, 6.9588) (0.6189, 6.9675) knots 0 0 0 0 1 1 1 1
  spline S593 degree 3 poles (0.6189, 6.9675) (0.5807, 6.9753) (0.5426, 6.9857) (0.5348, 6.99) knots 0 0 0 0 1 1 1 1
  spline S594 degree 3 poles (0.5348, 6.99) (0.5148, 7.0004) (0.4879, 7.0039) (0.324, 7.0152) knots 0 0 0 0 1 1 1 1
  spline S595 degree 3 poles (0.324, 7.0152) (0.2477, 7.0204) (0.1696, 7.023) (0.1505, 7.0195) knots 0 0 0 0 1 1 1 1
  spline S596 degree 3 poles (0.1505, 7.0195) (0.1314, 7.0169) (0.0438, 7.0117) (-0.0447, 7.0074) knots 0 0 0 0 1 1 1 1
  spline S597 degree 3 poles (-0.0447, 7.0074) (-0.1661, 7.0013) (-0.2138, 6.9961) (-0.2398, 6.9848) knots 0 0 0 0 1 1 1 1
  spline S598 degree 3 poles (-0.2398, 6.9848) (-0.2589, 6.9762) (-0.2902, 6.9623) (-0.3092, 6.9545) knots 0 0 0 0 1 1 1 1
  spline S599 degree 3 poles (-0.3092, 6.9545) (-0.4281, 6.9033) (-0.5521, 6.8365) (-0.5903, 6.8018) knots 0 0 0 0 1 1 1 1
  spline S600 degree 3 poles (-0.5903, 6.8018) (-0.638, 6.7584) (-0.6831, 6.748) (-0.7082, 6.7732) knots 0 0 0 0 1 1 1 1
  spline S601 degree 3 poles (-0.7082, 6.7732) (-0.7247, 6.7897) (-0.7646, 6.9042) (-0.7646, 6.9345) knots 0 0 0 0 1 1 1 1
  spline S602 degree 3 poles (-0.7646, 6.9345) (-0.7646, 6.9623) (-0.8999, 7.2416) (-0.9468, 7.3101) knots 0 0 0 0 1 1 1 1
  spline S603 degree 3 poles (-0.9468, 7.3101) (-0.998, 7.3847) (-1.0873, 7.4628) (-1.1593, 7.4957) knots 0 0 0 0 1 1 1 1
  spline S604 degree 3 poles (-1.1593, 7.4957) (-1.2591, 7.5417) (-1.3154, 7.553) (-1.443, 7.553) knots 0 0 0 0 1 1 1 1
  spline S605 degree 3 poles (-1.443, 7.553) (-1.5705, 7.553) (-1.5696, 7.553) (-1.7466, 7.5001) knots 0 0 0 0 1 1 1 1
  spline S606 degree 3 poles (-1.7466, 7.5001) (-1.8949, 7.455) (-1.9764, 7.376) (-2.0692, 7.1852) knots 0 0 0 0 1 1 1 1
  spline S607 degree 3 poles (-2.0692, 7.1852) (-2.1013, 7.1193) (-2.1039, 7.1089) (-2.1074, 7.023) knots 0 0 0 0 1 1 1 1
  spline S608 degree 3 poles (-2.1074, 7.023) (-2.11, 6.9501) (-2.1065, 6.9068) (-2.0883, 6.8079) knots 0 0 0 0 1 1 1 1
  spline S609 degree 3 poles (-2.0883, 6.8079) (-2.0684, 6.7003) (-2.0588, 6.67) (-2.0181, 6.5832) knots 0 0 0 0 1 1 1 1
  spline S610 degree 3 poles (-2.0181, 6.5832) (-1.9686, 6.4809) (-1.9599, 6.4401) (-1.9842, 6.4305) knots 0 0 0 0 1 1 1 1
  spline S611 degree 3 poles (-1.9842, 6.4305) (-1.992, 6.4279) (-2.0623, 6.4253) (-2.1412, 6.4253) knots 0 0 0 0 1 1 1 1
  spline S612 degree 3 poles (-2.1412, 6.4253) (-2.2948, 6.4253) (-2.4231, 6.4106) (-2.5194, 6.382) knots 0 0 0 0 1 1 1 1
  spline S613 degree 3 poles (-2.5194, 6.382) (-2.6547, 6.3421) (-2.7467, 6.3117) (-2.7814, 6.2952) knots 0 0 0 0 1 1 1 1
  spline S614 degree 3 poles (-2.7814, 6.2952) (-2.7909, 6.2909) (-2.8161, 6.2805) (-2.8378, 6.2709) knots 0 0 0 0 1 1 1 1
  spline S615 degree 3 poles (-2.8378, 6.2709) (-2.8595, 6.2623) (-2.9098, 6.2336) (-2.9505, 6.2067) knots 0 0 0 0 1 1 1 1
  spline S616 degree 3 poles (-2.9505, 6.2067) (-2.9913, 6.1807) (-3.0538, 6.1426) (-3.0893, 6.1226) knots 0 0 0 0 1 1 1 1
  spline S617 degree 3 poles (-3.0893, 6.1226) (-3.1934, 6.0645) (-3.2134, 6.0523) (-3.2515, 6.0237) knots 0 0 0 0 1 1 1 1
  spline S618 degree 3 poles (-3.2515, 6.0237) (-3.2723, 6.0081) (-3.3201, 5.9743) (-3.3591, 5.9483) knots 0 0 0 0 1 1 1 1
  spline S619 degree 3 poles (-3.3591, 5.9483) (-3.3973, 5.9222) (-3.4753, 5.865) (-3.5326, 5.8225) knots 0 0 0 0 1 1 1 1
  spline S620 degree 3 poles (-3.5326, 5.8225) (-3.5907, 5.7791) (-3.6592, 5.7297) (-3.6852, 5.7123) knots 0 0 0 0 1 1 1 1
  spline S621 degree 3 poles (-3.6852, 5.7123) (-3.772, 5.6542) (-3.7911, 5.636) (-3.7989, 5.6074) knots 0 0 0 0 1 1 1 1
  spline S622 degree 3 poles (-3.7989, 5.6074) (-3.8093, 5.5701) (-3.7989, 5.5527) (-3.7624, 5.5458) knots 0 0 0 0 1 1 1 1
  spline S623 degree 3 poles (-3.7624, 5.5458) (-3.746, 5.5423) (-3.7208, 5.5345) (-3.7078, 5.5276) knots 0 0 0 0 1 1 1 1
  spline S624 degree 3 poles (-3.7078, 5.5276) (-3.6948, 5.5206) (-3.6757, 5.5145) (-3.6662, 5.5137) knots 0 0 0 0 1 1 1 1
  spline S625 degree 3 poles (-3.6662, 5.5137) (-3.6297, 5.5128) (-3.5707, 5.4746) (-3.5386, 5.4321) knots 0 0 0 0 1 1 1 1
  spline S626 degree 3 poles (-3.5386, 5.4321) (-3.5204, 5.4079) (-3.497, 5.3853) (-3.4866, 5.381) knots 0 0 0 0 1 1 1 1
  spline S627 degree 3 poles (-3.4866, 5.381) (-3.3556, 5.3281) (-3.301, 5.3029) (-3.2836, 5.2873) knots 0 0 0 0 1 1 1 1
  spline S628 degree 3 poles (-3.2836, 5.2873) (-3.2741, 5.2786) (-3.2585, 5.2717) (-3.2498, 5.2717) knots 0 0 0 0 1 1 1 1
  spline S629 degree 3 poles (-3.2498, 5.2717) (-3.2411, 5.2717) (-3.2281, 5.2656) (-3.2203, 5.2587) knots 0 0 0 0 1 1 1 1
  spline S630 degree 3 poles (-3.2203, 5.2587) (-3.2125, 5.2517) (-3.1847, 5.2309) (-3.1587, 5.2136) knots 0 0 0 0 1 1 1 1
  spline S631 degree 3 poles (-3.1587, 5.2136) (-3.0971, 5.1736) (-3.0286, 5.119) (-2.9341, 5.0375) knots 0 0 0 0 1 1 1 1
  spline S632 degree 3 poles (-2.9341, 5.0375) (-2.8933, 5.0019) (-2.8282, 4.9533) (-2.7901, 4.929) knots 0 0 0 0 1 1 1 1
  spline S633 degree 3 poles (-2.7901, 4.929) (-2.7519, 4.9056) (-2.7016, 4.8718) (-2.6773, 4.8536) knots 0 0 0 0 1 1 1 1
  spline S634 degree 3 poles (-2.6773, 4.8536) (-2.6539, 4.8354) (-2.6305, 4.8206) (-2.627, 4.8206) knots 0 0 0 0 1 1 1 1
  spline S635 degree 3 poles (-2.627, 4.8206) (-2.6226, 4.8206) (-2.5897, 4.7998) (-2.5533, 4.7746) knots 0 0 0 0 1 1 1 1